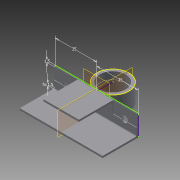
# Autodesk Inventor part: KisCsapagyHaz
Saved by Autodesk Inventor 2015 (Build 190159000, 159)
## iProperties
Created: 2014-09-27
Part Number: KisCsapagyHaz
Material: Generic
Document SubType Name: Modeling
Designer: laca
Density: 1 g/cm^3
Appearance: Default
Mass: 9.10248 g
Surface Area: 112.393 cm^2
Volume: 9.10248 cm^3
Author: laca
Autodesk Inventor part; units mm, degrees
ref_plane "YZ Plane" through (0, 0, 0) normal (1, 0, 0) x (0, 1, 0)
ref_plane "XZ Plane" through (0, 0, 0) normal (0, 1, 0) x (-1, 0, 0)
ref_plane "XY Plane" through (0, 0, 0) normal (0, 0, 1) x (1, 0, 0)
sketch "Sketch1" plane through (0, 0, 0) normal (0, 1, 0) x (-1, 0, 0)
  circle A0 centre (0, 0) radius 10.5
  circle A1 centre (0, 0) radius 13.5
  dimension "d0" = 21
  dimension "d1" = 3
  constraints: 2 centre point, 2 coincident
  measures "d0" diameter of A0
  measures "d1" radial gap between concentric circles of A1 A0
extrude "Extrusion1" add sketch "Sketch1" along normal blind 15
sketch "Sketch2" plane through (0, 15, 0) normal (0, 1, 0) x (1, 0, 0)
  circle A0 centre (0, 0) radius 11
  circle A1 centre (0, 0) radius 10.5
  dimension "d4" = 22
  dimension "d5" = 21
  constraints: 2 centre point, 2 coincident
  measures "d4" diameter of A0
  measures "d5" diameter of A1
extrude "Extrusion2" cut sketch "Sketch2" against normal blind 6
sketch "Sketch3" plane through (0, 15, 0) normal (0, 1, 0) x (1, 0, 0)
  line L0 (0, 0) -> (0, -13.5)
  circle A0 centre (0, 0) radius 13.5 projected
  constraints: 2 end point, 1 vertical, 1 vertical alignment, 1 other
ref_plane "Work Plane1" through (0, 15, 13.5) normal (0, 0, 1) x (1, 0, 0)
sketch "Sketch4" plane through (0, 15, 13.5) normal (0, 0, 1) x (1, 0, 0)
  line L0 (0, -15) -> (35, -15)
  line L1 (35, -15) -> (35, 0)
  line L2 (35, 0) -> (0, 0)
  line L3 (0, 0) -> (0, -15)
  line L4 (0, -15) -> (-35, -15)
  line L5 (-35, -15) -> (-35, 0)
  line L6 (-35, 0) -> (0, 0)
  line L7 (0, 0) -> (0, -15)
  line L8 (-35, 0) -> (35, 0)
  line L9 (35, 0) -> (35, 1.5)
  line L10 (35, 1.5) -> (-35, 1.5)
  line L11 (-35, 1.5) -> (-35, 0)
  line L12 (-35, -15) -> (35, -15)
  line L13 (35, -15) -> (35, -16.5)
  line L14 (35, -16.5) -> (-35, -16.5)
  line L15 (-35, -16.5) -> (-35, -15)
  dimension "d8" = 35
  dimension "d9" = 35
  dimension "d10" = 1.5
  dimension "d11" = 1.5
  constraints: 32 end point, 8 parallel, 4 horizontal, 4 perpendicular, 1 point on line
  measures "d8" distance of L5.end L6.end
  measures "d9" distance of L1.end L2.end
  measures "d10" distance between parallel lines of L6 L10
  measures "d11" distance between parallel lines of L14 L4
extrude "Extrusion3" add sketch "Sketch4" along normal blind 1.5
extrude "Extrusion4" add sketch "Sketch4" along normal blind 30 contours L0 L13 L14 L15 L4 | L6 L11 L10 L9 L2
fillet "Fillet1" radius 1 4 edges at (0, 15, 15) (0, 0, 15) (0, -1.5, 13.5) (0, 16.5, 13.5)
sketch "Sketch5" plane through (-35, 16.5, 43.5) normal (0, 1, 0) x (1, 0, 0)
  line L0 (0, 29) -> (0, 0) projected
  line L1 (70, 0) -> (0, 0) projected
  line L2 (0, 29) -> (20, 29)
  line L3 (20, 29) -> (20, 0)
  line L4 (20, 0) -> (0, 0)
  line L5 (0, 0) -> (0, 29)
  point P0 (35, 43.5)
  point P1 (70, 28.5)
  dimension "d28" = 20
  dimension "d29" = 29
  constraints: 8 end point, 2 parallel, 1 horizontal, 1 perpendicular, 1 point on line
  measures "d28" distance of L2.start L2.end
  measures "d29" distance of L4.end L2.start
extrude "Extrusion5" cut sketch "Sketch5" against normal blind 10
sketch "Sketch6" plane through (0, 15, 13.5) normal (0, 0, -1) x (-1, 0, 0)
  circle A0 centre (-25, -7.5) radius 2.5
  circle A1 centre (25, -7.5) radius 2.5
  line L0 (-35, -15.5) -> (-35, 0.5) projected
  line L1 (35, 0.5) -> (35, -15.5) projected
  line L2 (-35, 0) -> (35, 0) projected
  point P0 (0, -15)
  point P1 (-15, 0)
  dimension "d20" = 5
  dimension "d21" = 5
  dimension "d22" = 10
  dimension "d23" = 10
  dimension "d24" = 7.5
  constraints: 2 centre point, 1 horizontal alignment
  measures "d20" diameter of A0
  measures "d21" diameter of A1
  measures "d22" distance from line of L0 A0.centre
  measures "d23" distance from line of L1 A1.centre
  measures "d24" distance from line of L2 A1.centre
extrude "Extrusion6" cut sketch "Sketch6" against normal blind 10
ref_plane "Work Plane2" through (0, 15, 0) normal (1, 0, 0) x (0, 0, 1)
mirror "Mirror1" about plane through (0, 15, 0) normal (1, 0, 0) of "Extrusion5"
equation "\"d11\" = d10"
body "Solid1"
